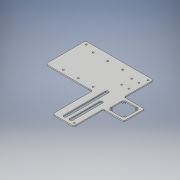
# Autodesk Inventor part: ThirdLayer
Saved by Autodesk Inventor 2018 (Build 220112000, 112)
## iProperties
Created: 2019-10-01
Part Number: ThirdLayer
Material: Generic
Document SubType Name: Modeling
Designer: anirudh
Density: 1 g/cm^3
Appearance: Default
Author: anirudh
Autodesk Inventor part; units mm, degrees
ref_plane "YZ Plane" through (0, 0, 0) normal (1, 0, 0) x (0, 1, 0)
ref_plane "XZ Plane" through (0, 0, 0) normal (0, 1, 0) x (-1, 0, 0)
ref_plane "XY Plane" through (0, 0, 0) normal (0, 0, 1) x (1, 0, 0)
sketch "Sketch1" plane through (0, 0, 0) normal (0, 1, 0) x (-1, 0, 0)
  line L0 (0, 0) -> (45, 0)
  line L1 (45, 0) -> (14.87, 0)
  line L2 (14.87, -170.18) -> (56.523, -170.18)
  line L3 (144.78, -163.83) -> (144.78, -85.18)
  line L4 (144.78, -85.18) -> (45, -85.18)
  line L5 (144.78, -163.83) -> (144.78, -170.18)
  line L6 (113.657, -170.18) -> (144.78, -170.18)
  line L7 (144.78, -170.18) -> (0, -170.18)
  line L8 (45, 0) -> (45, -85.18)
  circle A0 centre (5.08, -6.35) radius 1.75
  circle A1 centre (5.08, -163.83) radius 1.75
  circle A2 centre (137.16, -163.83) radius 1.75
  circle A3 centre (83.48, -93.35) radius 1.75
  circle A4 centre (83.48, -156.35) radius 1.75
  line L9 (-36.027, -96.0808) -> (-36.027, -97.5854)
  line L10 (-39.0316, -99.0854) -> (-39.0316, -71.0946)
  line L11 (-8.0362, -74.0992) -> (-8.0362, -72.5946)
  line L12 (-8.0362, -72.5946) -> (-8.0362, -74.0992)
  line L13 (-36.027, -68.09) -> (-8.0362, -68.09)
  arc A5 (-36.027, -96.0808) -> (-39.0316, -99.0854) centre (-36.027, -99.0854) ccw
  arc A6 (-8.0362, -68.09) -> (-11.0408, -71.0946) centre (-8.0362, -71.0946) ccw
  arc A7 (-36.027, -97.5854) -> (-34.527, -99.0854) centre (-36.027, -99.0854) ccw
  arc A8 (-36.027, -97.5854) -> (-34.527, -99.0854) centre (-36.027, -99.0854) ccw
  arc A9 (-8.0362, -72.5946) -> (-9.5362, -71.0946) centre (-8.0362, -71.0946) ccw
  arc A10 (-8.0362, -72.5946) -> (-9.5362, -71.0946) centre (-8.0362, -71.0946) ccw
  arc A11 (-8.0362, -74.0992) -> (-5.0316, -71.0946) centre (-8.0362, -71.0946) ccw
  line L14 (-5.0316, -99.0854) -> (-5.0316, -71.0946)
  line L15 (-8.0362, -102.09) -> (-36.027, -102.09)
  line L16 (-36.027, -102.09) -> (-8.0362, -102.09)
  arc A12 (-9.5362, -99.0854) -> (-8.0362, -97.5854) centre (-8.0362, -99.0854) ccw
  arc A13 (-9.5362, -99.0854) -> (-8.0362, -97.5854) centre (-8.0362, -99.0854) ccw
  arc A14 (-34.527, -71.0946) -> (-36.027, -72.5946) centre (-36.027, -71.0946) ccw
  arc A15 (-34.527, -71.0946) -> (-36.027, -72.5946) centre (-36.027, -71.0946) ccw
  line L17 (-8.0362, -97.5854) -> (-8.0362, -96.0808)
  arc A16 (-5.0316, -99.0854) -> (-8.0362, -96.0808) centre (-8.0362, -99.0854) ccw
  arc A17 (-5.0316, -99.0854) -> (-8.0362, -96.0808) centre (-8.0362, -99.0854) ccw
  line L18 (-8.0362, -97.5854) -> (-8.0362, -96.0808)
  line L19 (-34.527, -71.0946) -> (-33.0224, -71.0946)
  arc A18 (-33.0224, -71.0946) -> (-36.027, -68.09) centre (-36.027, -71.0946) ccw
  arc A19 (-39.0316, -71.0946) -> (-36.027, -74.0992) centre (-36.027, -71.0946) ccw
  arc A20 (-39.0316, -71.0946) -> (-36.027, -74.0992) centre (-36.027, -71.0946) ccw
  arc A21 (-33.0224, -71.0946) -> (-36.027, -68.09) centre (-36.027, -71.0946) ccw
  line L20 (-11.0408, -71.0946) -> (-9.5362, -71.0946)
  line L21 (-9.5362, -71.0946) -> (-11.0408, -71.0946)
  line L22 (-36.027, -97.5854) -> (-36.027, -96.0808)
  arc A22 (-36.027, -96.0808) -> (-39.0316, -99.0854) centre (-36.027, -99.0854) ccw
  line L23 (-34.527, -99.0854) -> (-33.0224, -99.0854)
  line L24 (-34.527, -99.0854) -> (-33.0224, -99.0854)
  arc A23 (-36.027, -102.09) -> (-33.0224, -99.0854) centre (-36.027, -99.0854) ccw
  line L25 (-11.0408, -99.0854) -> (-9.5362, -99.0854)
  line L26 (-11.0408, -99.0854) -> (-9.5362, -99.0854)
  arc A24 (-11.0408, -99.0854) -> (-8.0362, -102.09) centre (-8.0362, -99.0854) ccw
  line L27 (-36.027, -74.0992) -> (-36.027, -72.5946)
  line L28 (-36.027, -72.5946) -> (-36.027, -74.0992)
  line L29 (-36.027, -99.0854) -> (-23.327, -99.0854) construction
  line L30 (-36.027, -99.0854) -> (-27.137, -99.0854) construction
  arc A25 (-44.0632, -105.3716) -> (-42.3132, -107.1216) centre (-42.3132, -105.3716) ccw
  arc A26 (-42.3132, -63.0584) -> (-44.0632, -64.8084) centre (-42.3132, -64.8084) ccw
  line L31 (-42.3132, -63.0584) -> (0, -63.0584)
  line L32 (0, -107.1216) -> (-42.3132, -107.1216)
  line L33 (-44.0632, -105.3716) -> (-44.0632, -64.8084)
  line L34 (0, -170.18) -> (0, -107.1216)
  line L35 (0, -63.0584) -> (0, 0)
  circle A27 centre (10.16, -127.8558) radius 1.5
  circle A28 centre (10.16, -149.4458) radius 1.5
  circle A29 centre (25.4, -149.4458) radius 1.5
  circle A30 centre (25.4, -127.8558) radius 1.4986
  point P0 (-2.54, 0.1)
  dimension "d3" = 3.5
  dimension "d5" = 3.5
  dimension "d6" = 3.5
  dimension "d9" = 3
  dimension "d10" = 3
  dimension "d11" = 3
  dimension "d12" = 2.9972
  constraints: 72 end point, 44 point on circle, 31 centre point, 9 coincident, 8 tangent, 6 horizontal, 6 perpendicular, 5 collinear, 3 vertical
  measures "d3" diameter of A1
  measures "d5" diameter of A3
  measures "d6" diameter of A4
  measures "d9" diameter of A27
  measures "d10" diameter of A28
  measures "d11" diameter of A29
  measures "d12" diameter of A30
extrude "Extrusion1" add sketch "Sketch1" along normal blind 2.286
fillet "Fillet1" radius 3.175 8 edges at (-45, 1.143, 0) (0, 1.143, 0) (0, 1.143, -63.0584) (0, 1.143, -107.1216) (-45, 1.143, -85.18) (-144.78, 1.143, -85.18) (-144.78, 1.143, -170.18) (0, 1.143, -170.18)
sketch "Sketch2" plane through (0, 2.286, 0) normal (0, 1, 0) x (1, 0, 0)
  circle A0 centre (-51.7938, 156.5362) radius 1.75
  circle A1 centre (-115.1662, 156.5362) radius 1.75
  circle A2 centre (-115.1662, 93.1638) radius 1.65
  circle A3 centre (-115.1662, 93.1638) radius 1.75
  circle A4 centre (-51.7938, 93.1638) radius 1.65
  circle A5 centre (-51.7938, 93.1638) radius 1.75
  line L0 (-144.78, 167.005) -> (-144.78, 88.355) projected
  line L1 (0, 110.2966) -> (0, 167.005) projected
  circle A6 centre (-83.48, 93.35) radius 1.75 projected
  circle A7 centre (-83.48, 156.35) radius 1.75 projected
  point P0 (0, 0)
  dimension "d17" = 3.5
  dimension "d18" = 3.5
  dimension "d19" = 3.5
  dimension "d20" = 3.5
  constraints: 6 centre point, 4 coincident
  measures "d17" diameter of A0
  measures "d18" diameter of A1
  measures "d19" diameter of A3
  measures "d20" diameter of A5
extrude "Extrusion2" cut sketch "Sketch2" against normal blind 25.4 contours A0 | A1 | A2 | A3 | A4 | A5
sketch "Sketch3" plane through (0, 2.286, 0) normal (0, 1, 0) x (1, 0, 0)
  circle A0 centre (-5.08, 6.35) radius 1.75 projected
  arc A1 (-17.78, 9.525) -> (-11.43, 9.525) centre (-14.605, 9.525) ccw
  arc A2 (-30.48, 9.525) -> (-24.13, 9.525) centre (-27.305, 9.525) ccw
  arc A3 (-11.43, 73.025) -> (-17.78, 73.025) centre (-14.605, 73.025) ccw
  arc A4 (-24.13, 98.425) -> (-30.48, 98.425) centre (-27.305, 98.425) ccw
  line L0 (-30.48, 9.525) -> (-30.48, 98.425)
  line L1 (-24.13, 98.425) -> (-24.13, 9.525)
  line L2 (-17.78, 9.525) -> (-17.78, 73.025)
  line L3 (-11.43, 73.025) -> (-11.43, 9.525)
  point P0 (0, 0)
  constraints: 8 end point, 8 point on circle, 4 centre point, 3 parallel, 1 tangent, 1 vertical
extrude "Extrusion3" cut sketch "Sketch3" against normal blind 25.4 contours L2 A3 L3 A1 | L0 A4 L1 A2
body "Solid1"
